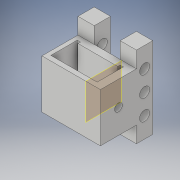
# Autodesk Inventor part: Objektträgerhalter 2 6,15mm
Saved by Autodesk Inventor 2018.3 (Build 223284000, 284)
## iProperties
Created: 2018-10-11
Part Number: Objektträgerhalter 2 6,15mm
Material: Generisch
Document SubType Name: Modeling
Designer: pgmadmin
Density: 1 g/cm^3
Appearance: Vorgabe
Author: pgmadmin
Autodesk Inventor part; units mm, degrees
ref_plane "YZ Plane" through (0, 0, 0) normal (1, 0, 0) x (0, 1, 0)
ref_plane "XZ Plane" through (0, 0, 0) normal (0, 1, 0) x (-1, 0, 0)
ref_plane "XY Plane" through (0, 0, 0) normal (0, 0, 1) x (1, 0, 0)
sketch "Skizze1" plane through (0, 0, 0) normal (0, 0, 1) x (1, 0, 0)
  line L0 (-14.1284, 0) -> (-14.1284, 16.2)
  line L1 (-14.1284, 16.2) -> (-12.1284, 16.2)
  line L2 (-12.1284, 16.2) -> (-12.1284, 1.6)
  line L3 (-12.1284, 1.6) -> (12.3716, 1.6)
  line L4 (12.3716, 1.6) -> (12.3716, 16.2)
  line L5 (12.3716, 16.2) -> (14.3716, 16.2)
  line L6 (14.3716, 16.2) -> (14.3716, 0)
  line L7 (14.3716, 0) -> (-14.1284, 0)
  line L8 (-16.6284, 19.2) -> (19.3716, 19.2)
  line L9 (19.3716, 19.2) -> (19.3716, -3)
  line L10 (19.3716, -3) -> (-16.6284, -3)
  line L11 (-16.6284, -3) -> (-16.6284, 19.2)
  line L12 (-12.1284, 14.7) -> (12.3716, 14.7)
  point P0 (0, 0)
  dimension "d1" = 2
  dimension "d3" = 2
  dimension "d4" = 1.6
  dimension "d5" = 3
  dimension "d7" = 2.5
  dimension "d8" = 5
  dimension "d9" = 1.5
  dimension "d26" = 3
  dimension "d27" = 28.5
  dimension "d28" = 16.2
  constraints: 26 end point, 8 perpendicular, 4 point on line, 2 parallel, 1 horizontal, 1 vertical
  measures "d1" distance of L0.end L1.end
  measures "d3" distance of L4.end L5.end
  measures "d4" distance between parallel lines of L3 L7
  measures "d5" distance between parallel lines of L10 L7
  measures "d7" distance between parallel lines of L11 L0
  measures "d8" distance between parallel lines of L9 L6
  measures "d9" distance of L1.end L12.start
  measures "d26" distance between parallel lines of L8 L1
  measures "d27" distance of L6.end L0.start
  measures "d28" distance of L0.start L0.end
extrude "Extrusion1" add sketch "Skizze1" along normal blind 30
ref_plane "Arbeitsebene1" through (19.3716, -1, 28) normal (1, 0, 0) x (0, 0, -1)
sketch "Skizze5" plane through (19.3716, -1, 28) normal (1, 0, 0) x (0, 0, -1)
  circle A0 centre (13, 9.1) radius 2.4
  line L0 (13, 9.1) -> (-2, 9.1)
  line L1 (-2, 18.2) -> (-2, 0) projected
  line L2 (13, 9.1) -> (13, 20.2)
  line L3 (8, 20.2) -> (18, 20.2) projected
  line L4 (13, 9.1) -> (28, 9.1)
  point P0 (28, 1)
  dimension "d31" = 4.8
  dimension "d32" = 90
  dimension "d35" = 15
  constraints: 6 end point, 2 midpoint, 1 centre point, 1 collinear, 1 horizontal, 1 vertical
  measures "d31" diameter of A0
  measures "d32" angle of L2 L0
  measures "d35" distance between parallel lines of L1 L2
extrude "Extrusion5" cut sketch "Skizze5" against normal blind 10
sketch "Skizze6" plane through (-16.6284, 19.2, 0) normal (0, 1, 0) x (1, 0, 0)
  line L0 (36, -30) -> (0, -30) projected
  line L1 (36, -30) -> (26, -30)
  line L2 (26, -30) -> (26, 0)
  line L3 (26, 0) -> (36, 0)
  line L4 (36, 0) -> (36, -30)
  line L5 (0.0037, -30) -> (10.0037, -30)
  line L6 (10.0037, -30) -> (10.0037, 0)
  line L7 (10.0037, 0) -> (0.0037, 0)
  line L8 (0.0037, 0) -> (0.0037, -30)
  line L9 (26, -30) -> (36, -30)
  line L10 (36, -30) -> (36, -40)
  line L11 (36, -40) -> (26, -40)
  line L12 (26, -40) -> (26, -30)
  line L13 (26, 0) -> (36, 0)
  line L14 (36, 0) -> (36, 10)
  line L15 (36, 10) -> (26, 10)
  line L16 (26, 10) -> (26, 0)
  line L17 (0.0037, 0) -> (10.0037, 0)
  line L18 (10.0037, 0) -> (10.0037, 10)
  line L19 (10.0037, 10) -> (0.0037, 10)
  line L20 (0.0037, 10) -> (0.0037, 0)
  line L21 (0.0037, -30) -> (10.0037, -30)
  line L22 (10.0037, -30) -> (10.0037, -40)
  line L23 (10.0037, -40) -> (0.0037, -40)
  line L24 (0.0037, -40) -> (0.0037, -30)
  point P0 (16.6284, 0)
  dimension "d36" = 10
  dimension "d37" = 30
  dimension "d38" = 10
  dimension "d39" = 30
  dimension "d40" = 10
  dimension "d41" = 10
  dimension "d42" = 10
  dimension "d43" = 10
  dimension "d44" = 10
  dimension "d45" = 10
  dimension "d46" = 10
  dimension "d47" = 10
  constraints: 48 end point, 12 parallel, 6 horizontal, 6 perpendicular, 1 point on line
  measures "d36" distance of L2.end L3.end
  measures "d37" distance of L1.end L2.end
  measures "d38" distance of L7.end L6.end
  measures "d39" distance of L6.end L5.end
  measures "d40" distance of L10.end L11.end
  measures "d41" distance of L9.end L10.end
  measures "d42" distance of L15.end L14.end
  measures "d43" distance of L14.end L13.end
  measures "d44" distance of L19.end L18.end
  measures "d45" distance of L18.end L17.end
  measures "d46" distance of L22.end L23.end
  measures "d47" distance of L21.end L22.end
extrude "Extrusion7" add sketch "Skizze6" along normal blind 10
sketch "Skizze8" plane through (-16.6248, 19.2, 30) normal (-1, 0, 0) x (0, 0, 1)
  line L0 (-40, 0) -> (-40, 10) projected
  point P0 (-30, -19.2)
  point P1 (-27.5, 5)
  point P2 (-15, 5)
  point P3 (-2.5, 5)
  dimension "d52" = 12.5
  dimension "d53" = 12.5
  dimension "d54" = 12.5
  measures "d52" distance from line of point (-27.5, 5) L0
  measures "d53" distance of point (-27.5, 5) point (-15, 5)
  measures "d54" distance of point (-2.5, 5) point (-15, 5)
hole "Bohrung1" at (-16.6248, 24.2, 2.5) at (-16.6248, 24.2, 15) at (-16.6248, 24.2, 27.5) direction (1, 0, 0) diameter 6.15 end through all
